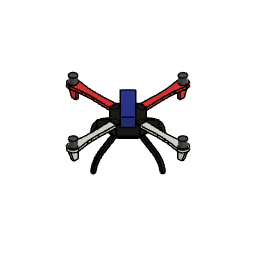
f450_quadcopter_lowpoly (Autodesk Fusion 360 design; units mm, degrees)
Autodesk Fusion 360 part; units mm, degrees
sketch "Sketch1" plane through (0, 0, 0) normal (0, 0, 1) x (1, 0, 0)
  line L0 (-137.0403, 426.6233) -> (-139.0124, 510.0377)
  line L1 (-139.0124, 510.0377) -> (-108.1035, 1318.302)
  line L2 (-108.1035, 1318.302) -> (-115.0262, 1611.1166)
  line L3 (-115.0262, 1611.1166) -> (-127.0111, 1780.42)
  line L4 (-127.0111, 1780.42) -> (-194.2816, 2220.2878)
  line L5 (0, 2250) -> (0, 0)
  line L6 (108.1035, 1318.302) -> (115.0262, 1611.1166)
  line L7 (115.0262, 1611.1166) -> (127.0111, 1780.42)
  line L8 (127.0111, 1780.42) -> (194.2816, 2220.2878)
  line L9 (139.0124, 510.0377) -> (108.1035, 1318.302)
  line L10 (137.0403, 426.6233) -> (139.0124, 510.0377)
  arc A0 (194.2816, 2220.2878) -> (-194.2816, 2220.2878) centre (0, 2250) ccw
  line L11 (-137.0403, 426.6233) -> (137.0403, 426.6233)
  dimension "d7" = 2250
  constraint coincident L5.end origin
  constraint vertical L5
  constraint symmetric L0.end L5 L9.start
  constraint symmetric L1.end L5 L6.start
  constraint symmetric L2.end L5 L6.end
  constraint symmetric L3.end L5 L7.end
  constraint symmetric L4.end L5 L8.end
  constraint symmetric L0.start L5 L10.start
  constraint coincident L8.end A0.start
  constraint coincident L4.end A0.end
  constraint coincident L5.start A0.centre
  constraint coincident L0.start L11.start
  constraint coincident L10.start L11.end
  measures "d7" distance of L5.start L5.end
extrude "Extrude1" add sketch "Sketch1" against normal blind 100 makes body 1
ref_plane "WorkPlane1" through (0, 469.9619, -50) normal (1, 0, 0) x (0, -1, 0)
sketch "Sketch3" plane through (0, 0, 0) normal (1, 0, 0) x (0, -1, 0)
  line L0 (2090, 100) -> (2090, 500)
  line L1 (2090, 500) -> (2260, 500)
  line L2 (2260, 500) -> (2410, 100)
  line L3 (2410, 100) -> (2090, 100)
  line L4 (2250, 100) -> (0, 100) construction
  dimension "d8" = 2250
  constraint vertical L0
  constraint perpendicular L0 L1
  constraint perpendicular L0 L3
  constraint midpoint L3 L4.start
  constraint parallel L3 L4
  measures "d8" distance of L4.start L4.end
extrude "Extrude2" add sketch "Sketch3" along normal mid plane 100 separate body makes body 2
pattern_circular "C-Pattern1" count 4 over 360 about axis through (0, 0, 1.75) along (0, 0, 1) of bodies 1 2 makes body 3 at (2253.3333, 50, -233.3333) makes body 4 at (-50, 2253.3333, -233.3333) makes body 5 at (-2253.3333, -50, -233.3333) makes body 6 at (-2073.6652, -42.337, 0) makes body 7 at (42.337, -2073.6652, 0) makes body 8 at (2073.6652, 42.337, 0)
sketch "Sketch6" plane through (0, 0, 0) normal (0, 0, 1) x (-1, 0, 0)
  line L0 (-510.0377, -139.0124) -> (-426.6233, -137.0403)
  line L1 (-426.6233, -137.0403) -> (-426.6233, 137.0403)
  line L2 (-426.6233, 137.0403) -> (-510.0377, 139.0124)
  line L3 (-510.0377, 139.0124) -> (-1318.302, 108.1035)
  line L4 (-1318.302, 108.1035) -> (-1611.1166, 115.0262)
  line L5 (-1611.1166, 115.0262) -> (-1780.42, 127.0111)
  line L6 (-1780.42, 127.0111) -> (-2220.2878, 194.2816)
  arc A0 (-2220.2878, 194.2816) -> (-2220.2878, -194.2816) centre (-2250, 0) ccw
  line L7 (-2220.2878, -194.2816) -> (-1780.42, -127.0111)
  line L8 (-1780.42, -127.0111) -> (-1611.1166, -115.0262)
  line L9 (-1611.1166, -115.0262) -> (-1318.302, -108.1035)
  line L10 (-1318.302, -108.1035) -> (-510.0377, -139.0124)
  line L11 (-615.7088, -134.9714) -> (-615.7088, 134.9714)
  line L12 (134.9714, -615.7088) -> (-134.9714, -615.7088)
  line L13 (615.7088, 134.9714) -> (615.7088, -134.9714)
  line L14 (-134.9714, 615.7088) -> (134.9714, 615.7088)
  line L15 (-134.9714, 615.7088) -> (-615.7088, 134.9714)
  line L16 (-615.7088, -134.9714) -> (-134.9714, -615.7088)
  line L17 (134.9714, -615.7088) -> (615.7088, -134.9714)
  line L18 (615.7088, 134.9714) -> (134.9714, 615.7088)
  dimension "d16" = 360
  constraint coincident L10 L11.start
  constraint coincident L3 L11.end
  constraint vertical L11
extrude "Extrude4" add sketch "Sketch6" along normal blind 20 separate body contours L0 L1 L2 L3 L10 L11 | L0 L1 L2 L3 L10 L12 L13 L14 L15 L16 L17 L18 makes body 9
extrude "Extrude5" add 1 faces at (-44.9905, 205.2363, 0) along direction (0, 0, -1) blind 400 separate body on bodies 9 makes body 10
sketch "Sketch7" plane through (0, 0, -400) normal (0, 0, -1) x (1, 0, 0)
  line L0 (-615.7088, -134.9714) -> (-134.9714, -615.7088)
  line L1 (-134.9714, -615.7088) -> (134.9714, -615.7088)
  line L2 (134.9714, -615.7088) -> (615.7088, -134.9714)
  line L3 (615.7088, -134.9714) -> (615.7088, 134.9714)
  line L4 (615.7088, 134.9714) -> (134.9714, 615.7088)
  line L5 (134.9714, 615.7088) -> (-134.9714, 615.7088)
  line L6 (-134.9714, 615.7088) -> (-615.7088, 134.9714)
  line L7 (-615.7088, 134.9714) -> (-615.7088, -134.9714)
  line L8 (-636.3961, 636.3961) -> (-424.2641, 848.5281)
  line L9 (-636.3961, 636.3961) -> (-848.5281, 424.2641)
  line L10 (848.5281, -424.2641) -> (424.2641, -848.5281)
  line L11 (0, 0) -> (424.2641, 424.2641) construction
  line L12 (424.2641, 424.2641) -> (636.3961, 212.132)
  line L13 (424.2641, 424.2641) -> (212.132, 636.3961)
  line L14 (0, 0) -> (-424.2641, -424.2641) construction
  line L15 (-424.2641, -424.2641) -> (-212.132, -636.3961)
  line L16 (-424.2641, -424.2641) -> (-636.3961, -212.132)
  line L17 (636.3961, 212.132) -> (636.3961, -212.132)
  line L18 (-636.3961, -212.132) -> (-636.3961, 212.132)
  line L19 (212.132, 636.3961) -> (-212.132, 636.3961)
  line L20 (-212.132, -636.3961) -> (212.132, -636.3961)
  line L21 (-848.5281, 424.2641) -> (-636.3961, 212.132)
  line L22 (212.132, -636.3961) -> (424.2641, -848.5281)
  line L23 (-424.2641, 848.5281) -> (-212.132, 636.3961)
  line L24 (636.3961, -212.132) -> (848.5281, -424.2641)
  dimension "d21" = 900
  dimension "d22" = 300
  dimension "d23" = 300
  dimension "d24" = 1800
  dimension "d25" = 1800
  dimension "d26" = 600
  dimension "d27" = 600
  dimension "d28" = 300
  dimension "d29" = 300
  constraint perpendicular L9 L21
  constraint perpendicular L6 L23
  constraint perpendicular L10 L21
  constraint coincident L11.start L14.start
  constraint perpendicular L11 L12
  constraint perpendicular L11 L13
  constraint perpendicular L14 L15
  constraint perpendicular L14 L16
  constraint coincident L17.end L23
  constraint parallel L3 L17
  constraint parallel L17 L18
  constraint parallel L5 L19
  constraint coincident L20.end L21
  constraint parallel L19 L20
  constraint collinear L21 L22
  constraint collinear L23 L24
  measures "d21" distance of L11.start L8.start
  measures "d22" distance of L8.start L8.end
  measures "d23" distance of L8.start L9.end
  measures "d24" distance of L9.end L10.end
  measures "d25" distance of L8.end L10.start
  measures "d26" distance of L11.start L11.end
  measures "d27" distance of L11.start L14.end
  measures "d28" distance of L14.end L15.end
  measures "d29" distance of L14.end L16.end
extrude "Extrude6" add sketch "Sketch7" along normal blind 20 separate body contours L0 L1 L2 L3 L4 L5 L6 L7 | L8 L9 L10 L12 L13 L15 L16 L17 L18 L19 L20 L21 L22 L23 L24 makes body 11
sketch "Sketch9" plane through (0, 0, 20) normal (0, 0, 1) x (-1, 0, 0)
  line L0 (134.9714, -615.7088) -> (615.7088, -134.9714)
  line L1 (615.7088, -134.9714) -> (615.7088, 134.9714)
  line L2 (615.7088, 134.9714) -> (134.9714, 615.7088)
  line L3 (134.9714, 615.7088) -> (-134.9714, 615.7088)
  line L4 (-134.9714, 615.7088) -> (-615.7088, 134.9714)
  line L5 (-615.7088, 134.9714) -> (-615.7088, -134.9714)
  line L6 (-615.7088, -134.9714) -> (-134.9714, -615.7088)
  line L7 (-134.9714, -615.7088) -> (134.9714, -615.7088)
  line L8 (225, -685) -> (-225, -685)
  line L9 (-225, -685) -> (-225, 685)
  line L10 (-225, 685) -> (225, 685)
  line L11 (225, 685) -> (225, -685)
  line L12 (225, -685) -> (-225, 685) construction
  line L13 (-225, -685) -> (225, 685) construction
  dimension "d32" = 450
  dimension "d33" = 1370
  constraint horizontal L8
  constraint perpendicular L8 L9
  constraint parallel L8 L10
  constraint parallel L9 L11
  constraint coincident L12 origin
  constraint coincident L13 origin
  measures "d32" distance of L9.end L10.end
  measures "d33" distance of L8.end L9.end
extrude "Extrude7" add sketch "Sketch9" along normal blind 370 separate body contours L0 L2 L3 L4 L6 L7 L9 L11 | L0 L6 L7 L8 L9 L11 | L2 L3 L4 L9 L10 L11 makes body 12
combine "Combine1" operation add target body 4 tool bodies 1
combine "Combine2" operation add target body 2 tool bodies 7
combine "Combine3" operation add target body 5 tool bodies 6
combine "Combine4" operation add target body 3 tool bodies 8
move_body "Move1" bodies 12 to x (0.707107, 0.707107, 0) y (-0.707107, 0.707107, 0) z (0, 0, 1) at (0, 0, 0)
sketch "Sketch10" plane through (0, 0, 0) normal (1, 0, 0) x (0, 1, 0)
  line L0 (600, -420) -> (350, -420)
  line L1 (350, -420) -> (350, -450)
  line L2 (350, -450) -> (600, -570)
  line L3 (600, -420) -> (1100, -720)
  line L4 (1033.1156, -831.4741) -> (600, -570)
  arc A0 (1375, -1350) -> (1033.1156, -831.4741) centre (660.0613, -1449.4152) ccw
  arc A1 (1475, -1350) -> (1100, -720) centre (701.8333, -1383.6111) ccw
  line L5 (1375, -1350) -> (1475, -1350)
  point P0 (1375, -1350)
  point P1 (1475, -1350)
  constraint perpendicular L0 L1
  constraint coincident P0 A0.start
  constraint tangent L4 A0
  constraint coincident P1 A1.start
  constraint tangent L3 A1
  constraint horizontal L5
extrude "Extrude8" add sketch "Sketch10" along normal mid plane 100 separate body makes body 13
pattern_circular "C-Pattern2" count 4 over 360 about axis through (0, 0, 1.75) along (0, 0, 1) of bodies 13 makes body 14 at (-766.6667, 50, -570) makes body 15 at (-50, -766.6667, -570) makes body 16 at (766.6667, -50, -570)
scale "Scale1" factor 0.1 about (1318.302, -108.1035, -100) bodies 10 2 15 4 9 13 3 5 14 11 16 12
move_body "Move2" bodies 13 9 12 5 15 14 10 3 11 16 4 2 to x (1, 0, 0) y (0, 1, 0) z (0, 0, 1) at (0, 0, 225)
move_body "Move3" bodies 3 4 16 9 15 14 10 11 5 12 13 2 to x (1, 0, 0) y (0, 1, 0) z (0, 0, 1) at (-1200, 105, 0)
move_body "Move4" bodies 14 4 16 2 12 13 9 11 10 3 5 15 to x (1, 0, 0) y (0, 1, 0) z (0, 0, 1) at (0, -7.6667, 0)
move_body "Move5" bodies 3 11 15 13 14 10 2 4 5 12 16 9 to x (1, 0, 0) y (0, 1, 0) z (0, 0, 1) at (13.5, 0, 0)
sketch "Sketch11" plane through (0, 0, 135) normal (0, 0, 1) x (-1, 0, 0)
  line L0 (51.032, 13.861) -> (42.6905, 13.6638)
  line L1 (42.6905, 13.6638) -> (42.6905, -13.7442)
  line L2 (42.6905, -13.7442) -> (51.032, -13.9414)
  line L3 (51.032, -13.9414) -> (131.8584, -10.8506)
  line L4 (131.8584, -10.8506) -> (161.1399, -11.5428)
  line L5 (161.1399, -11.5428) -> (178.0702, -12.7413)
  line L6 (178.0702, -12.7413) -> (222.057, -19.4684)
  arc A0 (222.057, -19.4684) -> (222.057, 19.388) centre (225.0282, -0.0402) ccw
  line L7 (222.057, 19.388) -> (178.0702, 12.6609)
  line L8 (178.0702, 12.6609) -> (161.1399, 11.4624)
  line L9 (161.1399, 11.4624) -> (131.8584, 10.7701)
  line L10 (131.8584, 10.7701) -> (51.032, 13.861)
  circle A1 centre (225.0282, -0.0402) radius 13.9
  dimension "d51" = 27.8
  constraint concentric A0 A1
  measures "d51" diameter of A1
extrude "Extrude9" add sketch "Sketch11" along normal blind 26.7 separate body contours A1 makes body 17
pattern_circular "C-Pattern3" count 4 over 360 about axis through (0, 0, 1.75) along (0, 0, 1) of bodies 17 makes body 18 at (-1.4242, -238.8591, 143.9) makes body 19 at (238.8591, -1.4242, 143.9) makes body 20 at (1.4242, 238.8591, 143.9)
equation "d7 = ( 4500 / 2 ) * 1 mm"
equation "d8 = ( 4500 / 2 ) * 1 mm"
named bodies: "Arm4", "Arm1", "Arm2", "Top", "Arm3", "Bottom", "Battery", "Leg1", "Leg2", "Leg3", "Leg4", "Motor2", "Motor3", "Motor4", "Motor1"
